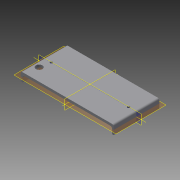
# Autodesk Inventor part: KarosserieDachTeil4
Saved by Autodesk Inventor 2015 (Build 190159000, 159)
## iProperties
Created: 2019-02-17
Part Number: KarosserieDachTeil4
Material: Generisch
Document SubType Name: Modeling
Designer: Boris
Density: 1 g/cm^3
Appearance: Vorgabe
Author: Boris
Autodesk Inventor part; units mm, degrees
sketch "Skizze1" plane through (0, 0, 0) normal (0, 0, 1) x (1, 0, 0)
  line L0 (-57, 28) -> (57, 28)
  line L1 (57, 28) -> (57, -28)
  line L2 (57, -28) -> (-57, -28)
  line L3 (-57, -28) -> (-57, 28)
  line L4 (0, -39.2) -> (0, 39.2) projected
  line L5 (-79.8, 0) -> (79.8, 0) projected
  circle A0 centre (-47.5, 0) radius 1.5
  circle A1 centre (47.5, 0) radius 1.5
  circle A2 centre (-50, -12.5) radius 4
  point P0 (0, 0)
  dimension "d0" = 114
  dimension "d1" = 56
  dimension "d2" = 3
  dimension "d3" = 47.5
  dimension "d4" = 8
  dimension "d5" = 40.5
  dimension "d6" = 7
  constraints: 8 end point, 3 centre point, 2 parallel, 1 horizontal, 1 perpendicular, 1 point on line, 1 symmetric about line, 3 other
  measures "d0" distance of L1.end L2.end
  measures "d1" distance of L0.end L1.end
  measures "d2" diameter of A0
  measures "d3" distance from line of A0.centre L4
  measures "d4" diameter of A2
  measures "d5" distance from line of L0 A2.centre
  measures "d6" distance from line of L3 A2.centre
extrude "Extrusion1" add sketch "Skizze1" along normal mid plane 11 contours L0 L4 L5 A0 L3 | L0 L1 L5 A1 L4 | L5 A0 L4 L2 L3 | L5 A1 L1 L2 L4
sketch "Skizze2" plane through (0, 0, -5.5) normal (0, 0, -1) x (-1, 0, 0)
  line L0 (57, -28) -> (57, 28) projected
  line L1 (-57, 28) -> (-57, -28) projected
  line L2 (55, -28) -> (55, 28)
  line L3 (-55, 28) -> (-55, -28)
  line L4 (55, -28) -> (-55, -28)
  line L5 (-55, 28) -> (55, 28)
  line L6 (-57, 28) -> (57, 28) projected
  point P0 (0, 0)
  dimension "d9" = 2
  dimension "d10" = 2
  constraints: 8 end point, 2 parallel, 1 collinear, 1 perpendicular
  measures "d9" distance between parallel lines of L0 L2
  measures "d10" distance between parallel lines of L1 L3
extrude "Extrusion2" cut sketch "Skizze2" against normal blind 8
fillet "Rundung1" radius 2 2 edges at (-57, 0, 5.5) (57, 0, 5.5)
fillet "Rundung2" radius 2 2 edges at (-55, 0, 2.5) (55, 0, 2.5)
